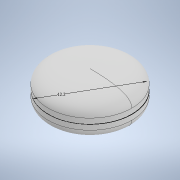
# Autodesk Inventor part: pillen
Saved by Autodesk Inventor 2020 (Build 240168000, 168)
## iProperties
Created: 2022-04-08
Part Number: pillen
Material: Generic
Document SubType Name: Modeling
Designer: Mic
Density: 1 g/cm^3
Appearance: Default
Author: Mic
Autodesk Inventor part; units mm, degrees
ref_plane "YZ Plane" through (0, 0, 0) normal (1, 0, 0) x (0, 1, 0)
ref_plane "XZ Plane" through (0, 0, 0) normal (0, 1, 0) x (-1, 0, 0)
ref_plane "XY Plane" through (0, 0, 0) normal (0, 0, 1) x (1, 0, 0)
sketch "Sketch1" plane through (0, 0, 0) normal (0, 1, 0) x (-1, 0, 0)
  circle A0 centre (0, 0) radius 6.1
  dimension "d0" = 12.2
  constraints: 1 centre point, 1 coincident
  measures "d0" diameter of A0
sketch "Sketch2" plane through (0, 0, 0) normal (0, 0, 1) x (1, 0, 0)
  line L0 (0, 0) -> (0, 2.7)
  line L1 (0, 0) -> (0, -2.7)
  line L2 (0, 0) -> (6.1265, 0)
  line L3 (6.1265, 0) -> (6.1265, 2.7)
  line L4 (6.1265, 2.7) -> (0, 2.7)
  line L5 (6.1265, 0.768) -> (6.1265, 2.7) construction
  line L6 (6.1265, 2.7) -> (0, 2.7) construction
  spline S0 degree 2 poles (6.1265, 0.768) (6.1265, 2.7) (0, 2.7) knots 1 1 1 2 2 2
  dimension "d1" = 2.7
  dimension "d2" = 2.7
  constraints: 10 end point, 3 perpendicular, 2 vertical, 1 coincident, 1 collinear, 1 horizontal, 1 point on line, 3 other
  measures "d1" distance of L0.start L0.end
  measures "d2" distance of L0.start L1.end
revolve "Revolution1" add sketch "Sketch2" angle 360 about axis through (0, 0, 0) along (0, 1, 0) contours L0 S0 L3 L2
mirror "Mirror1" about plane through (0, 0, 0) normal (0, -1, 0) of "Revolution1"
body "Solid1"
